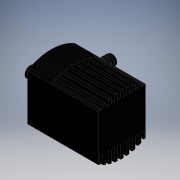
# Autodesk Inventor part: To Much Work, Motor
Saved by Autodesk Inventor 2016 (Build 200138000, 138)
## iProperties
Created: 2016-03-05
Part Number: To Much Work, Motor
Material: Generic
Document SubType Name: Modeling
Designer: Kenneth Daniel
Density: 1 g/cm^3
Appearance: Default
Author: Kenneth Daniel
Autodesk Inventor part; units mm, degrees
ref_plane "YZ Plane" through (0, 0, 0) normal (1, 0, 0) x (0, 1, 0)
ref_plane "XZ Plane" through (0, 0, 0) normal (0, 1, 0) x (-1, 0, 0)
sketch "Sketch1" plane through (0, 0, 0) normal (0, 1, 0) x (-1, 0, 0)
  line L0 (25.5, -21.35) -> (-25.5, -21.35)
  line L1 (-25.5, -21.35) -> (-25.5, 21.35)
  line L2 (-25.5, 21.35) -> (25.5, 21.35)
  line L3 (25.5, 21.35) -> (25.5, -21.35)
  line L4 (25.5, -21.35) -> (-25.5, 21.35) construction
  line L5 (-25.5, -21.35) -> (25.5, 21.35) construction
  point P0 (0, 0)
  dimension "d0" = 51
  dimension "d1" = 42.7
  constraints: 12 end point, 2 midpoint, 2 parallel, 1 horizontal, 1 perpendicular
  measures "d0" distance of L0.start L0.end
  measures "d1" distance of L0.end L1.end
extrude "Extrusion1" add sketch "Sketch1" along normal blind 34
sketch "Sketch2" plane through (-25.5, 0, -21.35) normal (-1, 0, 0) x (0, 0, 1)
  line L0 (42.7, 0) -> (0, 0) projected
  line L1 (42.7, 0) -> (42.7, 34) projected
  line L2 (0, 34) -> (42.7, 34) projected
  line L3 (0, 0) -> (0, 34) projected
  arc A0 (38.0522, 0) -> (38.0522, 34) centre (9.2864, 17) ccw
  line L4 (0, 34) -> (42.7, 34) construction
  line L5 (21.35, 34) -> (21.35, 0) construction
  arc A1 (4.6478, 34) -> (4.6478, 0) centre (33.4136, 17) ccw
  line L6 (0, 17) -> (42.7, 17) construction
  line L7 (42.7, 0) -> (0, 0) construction
  line L8 (9.5522, 34) -> (9.5522, 0) construction
  line L9 (9.5522, 34) -> (9.5522, 0)
  line L10 (0, 0) -> (0, 34) construction
  line L11 (0.0169, 18.0624) -> (9.5522, 18.0624) construction
  line L12 (9.5522, 15.937) -> (0, 15.937) construction
  line L13 (9.5522, 18.0624) -> (0.0169, 18.0624)
  line L14 (9.5522, 15.937) -> (0.0169, 15.937)
  line L15 (0.152, 20.1831) -> (9.5522, 20.1831)
  line L16 (0.4243, 22.3081) -> (9.5522, 22.3081)
  line L17 (0.8373, 24.4331) -> (9.5522, 24.4331)
  line L18 (1.3962, 26.5581) -> (9.5522, 26.5581)
  line L19 (2.1091, 28.6831) -> (9.5522, 28.6831)
  line L20 (2.9865, 30.8081) -> (9.5522, 30.8081)
  line L21 (4.0434, 32.9331) -> (9.5522, 32.9331)
  line L22 (0.1524, 13.812) -> (9.5522, 13.812)
  line L23 (0.4251, 11.687) -> (9.5522, 11.687)
  line L24 (0.8384, 9.562) -> (9.5522, 9.562)
  line L25 (1.3977, 7.437) -> (9.5522, 7.437)
  line L26 (2.1109, 5.312) -> (9.5522, 5.312)
  line L27 (2.9888, 3.187) -> (9.5522, 3.187)
  line L28 (4.0461, 1.062) -> (9.5522, 1.062)
  line L29 (9.5522, 34) -> (0, 34)
  line L30 (0, 34) -> (0, 0)
  line L31 (0, 0) -> (4.6478, 0)
  line L32 (42.7, 0) -> (42.7, 34) projected
  line L33 (42.7, 0) -> (42.7, 34)
  line L34 (42.7, 34) -> (9.5522, 34)
  line L35 (42.7, 0) -> (0, 0)
  line L36 (4.6478, 34) -> (4.0434, 32.9331)
  dimension "d4" = 28.5
  dimension "d5" = 1.0625
  dimension "d6" = 1.063
  dimension "d7" = 2.125
  dimension "d8" = 2.125
  dimension "d9" = 2.125
  dimension "d10" = 2.125
  dimension "d11" = 2.125
  dimension "d12" = 2.125
  dimension "d13" = 2.125
  dimension "d14" = 2.125
  dimension "d15" = 2.125
  dimension "d16" = 2.125
  dimension "d17" = 2.125
  dimension "d18" = 2.125
  dimension "d19" = 2.125
  dimension "d20" = 2.125
  dimension "d21" = 1.062
  dimension "d22" = 1.0669
  constraints: 56 end point, 9 perpendicular, 6 collinear, 6 horizontal, 5 point on line, 4 parallel, 3 point on circle, 3 symmetric about line, 2 vertical, 1 centre point, 1 midpoint, 41 other
  measures "d4" distance of A0.end L8.start
  measures "d5" distance of L6.start L11.start
  measures "d6" distance of L6.start L12.end
  measures "d7" distance of L15.start L11.start
  measures "d8" distance between parallel lines of L16 L15
  measures "d9" distance between parallel lines of L17 L16
  measures "d10" distance between parallel lines of L18 L17
  measures "d11" distance between parallel lines of L19 L18
  measures "d12" distance between parallel lines of L20 L19
  measures "d13" distance between parallel lines of L21 L20
  measures "d14" distance between parallel lines of L22 L12
  measures "d15" distance between parallel lines of L23 L22
  measures "d16" distance between parallel lines of L24 L23
  measures "d17" distance between parallel lines of L25 L24
  measures "d18" distance between parallel lines of L26 L25
  measures "d19" distance between parallel lines of L27 L26
  measures "d20" distance between parallel lines of L28 L27
  measures "d21" distance of L8.end L28.end
  measures "d22" distance of L21.end L8.start
extrude "Extrusion2" cut sketch "Sketch2" against normal through all contours L0 L3 A1 | L28 A1 L27 L9 | L9 L21 L36 L2 | A1 L3 L2 | L9 L20 A1 L21 | L26 A1 L25 L9 | A1 L15 L9 L13 | L14 L9 L22 A1 | L9 L18 A1 L19 | L24 A1 L23 L9 | A1 L17 L9 L16
sketch "Sketch3" plane through (-25.5, 0, 21.35) normal (-1, 0, 0) x (0, 0, 1)
  line L0 (-38.6566, 32.9331) -> (-33.1478, 32.9331)
  line L1 (-33.1478, 34) -> (-33.1478, 30.8081) projected
  line L2 (0, 34) -> (-33.1478, 34) projected
  line L3 (-38.0522, 34) -> (-33.1478, 34)
  line L4 (-33.1478, 34) -> (-33.1478, 32.9331)
  arc A0 (-38.0522, 34) -> (-38.6566, 32.9331) centre (-9.2864, 17) ccw projected
  line L5 (-38.0522, 34) -> (-38.0522, 34)
  line L6 (-38.0522, 34) -> (-38.6566, 32.9331)
  point P0 (-21.35, 0)
  constraints: 10 end point, 2 horizontal, 2 point on line, 1 collinear, 1 point on circle
extrude "Extrusion3" add sketch "Sketch3" against normal blind 51 contours L6 L3 L1 L0
sketch "Sketch4" plane through (-25.5, 0, 21.35) normal (0, 0, 1) x (1, 0, 0)
  line L0 (51, 34) -> (0, 34) projected
  line L1 (17, 34) -> (17, 0)
  line L2 (0, 0) -> (51, 0) projected
  line L3 (0, 30.8081) -> (51, 30.8081) projected
  line L4 (0, 28.6831) -> (51, 28.6831) projected
  line L5 (0, 26.5581) -> (51, 26.5581) projected
  line L6 (0, 24.4331) -> (51, 24.4331) projected
  line L7 (0, 22.3081) -> (51, 22.3081) projected
  line L8 (0, 20.1831) -> (51, 20.1831) projected
  line L9 (0, 18.0624) -> (51, 18.0624) projected
  line L10 (51, 15.937) -> (0, 15.937) projected
  line L11 (51, 0) -> (0, 0) projected
  line L12 (51, 0) -> (51, 34) projected
  line L13 (0, 34) -> (51, 34) projected
  line L14 (0, 0) -> (0, 34) projected
  line L15 (0, 13.812) -> (51, 13.812) projected
  line L16 (0, 11.687) -> (51, 11.687) projected
  line L17 (0, 9.562) -> (51, 9.562) projected
  line L18 (0, 7.437) -> (51, 7.437) projected
  line L19 (0, 5.312) -> (51, 5.312) projected
  line L20 (0, 3.187) -> (51, 3.187) projected
  line L21 (0, 1.062) -> (51, 1.062) projected
  line L22 (0, 32.9331) -> (51, 32.9331) projected
  line L23 (17, 34) -> (51, 34)
  line L24 (51, 34) -> (51, 0)
  line L25 (51, 1.062) -> (51, 3.187) projected
  line L26 (51, 0) -> (51, 1.062) projected
  line L27 (51, 0) -> (17, 0)
  line L28 (17, 1.062) -> (51, 1.062)
  line L29 (51, 3.187) -> (51, 5.312) projected
  line L30 (51, 3.187) -> (17, 3.187)
  line L31 (17, 5.312) -> (51, 5.312)
  line L32 (51, 5.312) -> (51, 7.437)
  line L33 (51, 7.437) -> (17, 7.437)
  line L34 (51, 7.437) -> (51, 9.562) projected
  line L35 (17, 9.562) -> (51, 9.562)
  line L36 (51, 9.562) -> (51, 11.687)
  line L37 (51, 11.687) -> (51, 13.812) projected
  line L38 (17, 11.687) -> (51, 11.687)
  line L39 (51, 11.687) -> (51, 13.812)
  line L40 (51, 13.812) -> (17, 13.812)
  line L41 (0, 13.812) -> (51, 13.812) projected
  line L42 (0, 15.937) -> (51, 15.937) projected
  line L43 (51, 15.937) -> (51, 18.0624) projected
  line L44 (17, 15.937) -> (51, 15.937)
  line L45 (51, 15.937) -> (51, 18.0624)
  line L46 (51, 18.0624) -> (17, 18.0624)
  line L47 (17, 20.1831) -> (51, 20.1831)
  line L48 (51, 22.3081) -> (17, 22.3081)
  line L49 (17, 24.4331) -> (51, 24.4331)
  line L50 (51, 26.5581) -> (17, 26.5581)
  line L51 (0, 26.5581) -> (51, 26.5581) projected
  line L52 (51, 28.6831) -> (51, 30.8081) projected
  line L53 (17, 28.6831) -> (51, 28.6831)
  line L54 (51, 28.6831) -> (51, 30.8081)
  line L55 (51, 30.8081) -> (17, 30.8081)
  line L56 (51, 30.8081) -> (51, 32.9331) projected
  line L57 (17, 32.9331) -> (51, 32.9331)
  point P0 (25.5, 0)
  dimension "d27" = 17
  constraints: 48 end point, 18 point on line, 7 collinear, 5 horizontal, 3 perpendicular, 2 vertical, 21 other
  measures "d27" distance of L23.start L0.end
extrude "Extrusion4" cut sketch "Sketch2" against normal blind 51 contours L0 A0 L1 | A0 L2 L1
sketch "Sketch5" plane through (25.5, 18.0624, -11.7978) normal (1, 0, 0) x (0, 0, -1)
  arc A0 (-28.5, 15.9376) -> (-28.5, -18.0624) centre (0.2657, -1.0624) ccw projected
  line L0 (-28.5, -18.0624) -> (-28.5, 15.9376)
  line L1 (-33.1478, -18.0624) -> (-33.1478, 15.9376) projected
  line L2 (-29.1017, -17.0004) -> (-28.5, -17.0004)
  line L3 (-30.1591, -14.8754) -> (-28.5, -14.8754)
  line L4 (-31.037, -12.7504) -> (-28.5, -12.7504)
  line L5 (-31.7501, -10.6254) -> (-28.5, -10.6254)
  line L6 (-32.3095, -8.5004) -> (-28.5, -8.5004)
  line L7 (-32.7227, -6.3754) -> (-28.5, -6.3754)
  line L8 (-32.9954, -4.2504) -> (-28.5, -4.2504)
  line L9 (-33.1309, -2.1254) -> (-28.5, -2.1254)
  line L10 (-33.131, 0) -> (-28.5, 0)
  line L11 (-32.9959, 2.1207) -> (-28.5, 2.1207)
  line L12 (-32.7235, 4.2457) -> (-28.5, 4.2457)
  line L13 (-32.3106, 6.3707) -> (-28.5, 6.3707)
  line L14 (-31.7516, 8.4957) -> (-28.5, 8.4957)
  line L15 (-31.0388, 10.6207) -> (-28.5, 10.6207)
  line L16 (-30.1613, 12.7457) -> (-28.5, 12.7457)
  line L17 (-29.1044, 14.8707) -> (-28.5, 14.8707)
  line L18 (-33.131, 0) -> (-28.5, 0)
  line L19 (-33.131, 0) -> (-28.5, 0)
  point P0 (-11.7978, -18.0624)
  point P1 (-33.1478, -12.7504)
  point P2 (-33.1478, -10.6254)
  point P3 (-33.1478, -8.5004)
  point P4 (-33.1478, -6.3754)
  point P5 (-33.1478, -4.2504)
  point P6 (-33.1478, -2.1254)
  point P7 (-33.1478, 0)
  point P8 (-33.1478, 2.1207)
  point P9 (-33.1478, 4.2457)
  point P10 (-33.1478, 6.3707)
  point P11 (-33.1478, 8.4957)
  point P12 (-33.1478, 10.6207)
  point P13 (-33.1478, 12.7457)
  point P14 (-33.1478, 14.8707)
  point P15 (-33.1478, -14.8754)
  point P16 (-33.1478, -17.0004)
  constraints: 36 end point, 15 horizontal, 2 collinear, 1 parallel, 37 other
extrude "Extrusion5" cut sketch "Sketch5" against normal blind 34 contours L17 L0 L16 A0 | L15 L0 L14 A0 | L13 L0 L12 A0 | L11 L0 L10 A0 | L0 L8 A0 L9 | L0 L6 A0 L7 | L0 L4 A0 L5 | L0 L2 A0 L3
sketch "Sketch6" plane through (0, 34, 0) normal (0, 1, 0) x (1, 0, 0)
  line L0 (-25.5, 16.7022) -> (25.5, 16.7022) construction
  line L1 (-18.54, 16.7022) -> (-18.54, -16.7022) construction
  line L2 (25.5, -16.7022) -> (-25.5, -16.7022) construction
  line L3 (-25.5, 16.7022) -> (-25.5, -16.7022) construction
  circle A0 centre (-18.54, 0) radius 3.9688 construction
  circle A1 centre (-18.54, 0) radius 5.5563 construction
  circle A2 centre (-18.54, 0) radius 3.5 construction
  circle A3 centre (-18.54, 0) radius 3.5
  circle A4 centre (-18.54, 0) radius 3.9688
  point P0 (0, 0)
  dimension "d32" = 6.96
  dimension "d33" = 7.9375
  dimension "d34" = 11.1125
  dimension "d35" = 7
  constraints: 5 centre point, 4 coincident, 2 end point, 2 point on line, 1 concentric, 1 midpoint, 1 vertical
  measures "d32" distance between parallel lines of L3 L1
  measures "d33" diameter of A0
  measures "d34" diameter of A1
  measures "d35" diameter of A2
extrude "Extrusion6" add sketch "Sketch6" along normal blind 20
ref_plane "Work Plane3" through (-18.54, 34, 0) normal (0, 0, -1) x (-1, 0, 0)
ref_plane "Work Plane1" through (-18.54, 34, 3.9688) normal (0, 0, -1) x (-1, 0, 0)
ref_plane "Work Plane2" through (-18.54, 34, -3.9688) normal (0, 0, -1) x (-1, 0, 0)
sketch "Sketch7" plane through (-18.54, 34, 0) normal (0, 0, -1) x (-1, 0, 0)
  line L0 (3.9688, 20) -> (-3.9688, 20) projected
  line L1 (-3.9688, 0) -> (3.9688, 0) projected
  line L2 (3.9688, 20) -> (-3.9688, 20) projected
  line L3 (-3.9688, 0) -> (3.9688, 0) projected
  line L4 (3.9688, 20) -> (-3.9688, 20) projected
  line L5 (3.5, 0) -> (3.5, 20) projected
  line L6 (3.5, 17.4442) -> (3.9688, 17.4442)
  arc A0 (3.9688, 18.1132) -> (3.5, 20) centre (-1.4093, 17.7787) ccw
  line L7 (3.9688, 0) -> (3.9688, 20) projected
  line L8 (3.9688, 18.1132) -> (3.5, 17.4442)
  line L9 (3.9688, 17.4442) -> (2.7369, 17.4442) construction
  arc A1 (3.9688, 15.5575) -> (3.5, 17.4442) centre (-1.4093, 15.2229) ccw
  line L10 (3.9688, 15.5575) -> (3.5, 14.8884)
  arc A2 (3.9688, 13.0017) -> (3.5, 14.8884) centre (-1.4093, 12.6671) ccw
  line L11 (3.9688, 13.0017) -> (3.5, 12.3326)
  arc A3 (3.9688, 10.4459) -> (3.5, 12.3326) centre (-1.4093, 10.1113) ccw
  line L12 (3.9688, 10.4459) -> (3.5, 9.7768)
  line L13 (3.5, 20) -> (3.5, 9.7768) construction
  line L14 (0, 20) -> (0, 0) construction
  point P0 (-18.54, -34)
  dimension "d38" = 2.5558
  dimension "d39" = 0
  dimension "d40" = 0
  dimension "d41" = 0
  constraints: 16 end point, 8 point on circle, 4 centre point, 3 point on line, 2 midpoint, 1 collinear, 1 perpendicular
  measures "d38" distance between parallel lines of L0 L6
  measures "d39" distance of A2.end L10.end
  measures "d40" distance of L11.end A3.end
  measures "d41" distance of L6.start A1.end
revolve "Revolution1" cut sketch "Sketch7" angle 360 about axis through (-18.54, 54, 0) along (0, -1, 0) contours L7 A0 L0
sketch "Sketch8" plane through (-18.54, 34, 0) normal (0, 0, -1) x (-1, 0, 0)
  line L0 (-3.9688, 18.1132) -> (3.9688, 18.1132) projected
  line L1 (-3.9688, 18.1132) -> (-3.5, 17.5638)
  line L2 (-3.5, 0) -> (-3.5, 20) projected
  line L3 (-3.9688, 0) -> (-3.9688, 18.1132) projected
  arc A0 (-3.5, 17.5638) -> (-3.9688, 16.0073) centre (-0.6147, 15.846) ccw
  line L4 (-3.9688, 15.6848) -> (-3.5, 15.1353)
  arc A1 (-3.5, 15.1353) -> (-3.9688, 13.7438) centre (-0.9417, 13.4988) ccw
  line L5 (-3.9688, 13.2539) -> (-3.5, 12.7044)
  arc A2 (-3.5, 12.7044) -> (-3.9688, 11.1551) centre (-0.6356, 10.9922) ccw
  line L6 (-3.9688, 10.8293) -> (-3.5, 10.2798)
  line L7 (-3.5, 20) -> (3.5, 20) construction
  line L8 (0, 20) -> (0, 6.8356) construction
  point P0 (-18.54, -34)
  constraints: 10 end point, 6 point on circle, 4 point on line, 3 centre point, 1 midpoint, 1 vertical, 7 other
revolve "Revolution2" cut sketch "Sketch8" angle 360 about axis through (-18.54, 54, 0) along (0, -1, 0) contours L1 A0 L3 | A1 L3 L4 | A2 L3 L5
sketch "Sketch9" plane through (-25.5, 18.0624, -21.3331) normal (-1, 0, 0) x (0, 0, 1)
  line L0 (9.5353, 14.8707) -> (4.0266, 14.8707) construction
  line L1 (9.5353, 14.8707) -> (9.5353, 15.9376) construction
  line L2 (4.631, 15.9376) -> (38.0353, 15.9376) construction
  line L3 (9.5353, 15.9376) -> (38.0353, -18.0624) construction
  line L4 (38.0353, -18.0624) -> (38.0353, 15.9376) construction
  line L5 (38.0353, 14.8707) -> (38.0353, 12.7457) construction
  line L6 (38.0353, 15.9376) -> (9.5353, -18.0624) construction
  line L7 (38.0353, -18.0624) -> (4.631, -18.0624) construction
  circle A0 centre (21.3331, -1.0624) radius 3.5 construction
  circle A1 centre (21.3331, -1.0624) radius 3.969 construction
  circle A2 centre (21.3331, -1.0624) radius 3.5
  circle A3 centre (21.3331, -1.0624) radius 3.969
  point P0 (21.3331, -18.0624)
  dimension "d44" = 7
  dimension "d45" = 7.938
  constraints: 8 end point, 4 centre point, 3 coincident, 3 point on line, 2 concentric, 1 collinear, 1 vertical
  measures "d44" diameter of A0
  measures "d45" diameter of A1
extrude "Extrusion7" add sketch "Sketch9" along normal blind 15
sketch "Sketch10" plane through (-25.5, 18.0624, -21.3331) normal (-1, 0, 0) x (0, 0, 1)
  line L0 (9.5353, 14.8707) -> (4.0266, 14.8707) construction
  line L1 (9.5353, 14.8707) -> (9.5353, 15.9376) construction
  line L2 (4.631, 15.9376) -> (38.0353, 15.9376) construction
  line L3 (9.5353, 15.9376) -> (38.0353, -18.0624) construction
  line L4 (38.0353, -18.0624) -> (38.0353, 15.9376) construction
  line L5 (38.0353, 15.9376) -> (9.5353, -18.0624) construction
  line L6 (13.0353, 15.9376) -> (13.0353, -18.0624) construction
  line L7 (34.5353, 15.9376) -> (34.5353, -18.0624) construction
  circle A0 centre (13.0353, 11.7622) radius 1.75
  circle A1 centre (34.5353, 11.7622) radius 1.75
  circle A2 centre (34.5353, -13.8869) radius 1.75
  circle A3 centre (13.0353, -13.8869) radius 1.75
  point P0 (21.3331, -18.0624)
  dimension "d48" = 3.5
  dimension "d49" = 3.5
  dimension "d50" = 3.5
  dimension "d51" = 3.5
  dimension "d52" = 3.5
  dimension "d53" = 3.5
  constraints: 12 end point, 12 point on line, 4 centre point, 3 vertical, 1 parallel
  measures "d48" distance of L1.end L6.start
  measures "d49" distance of L2.end L7.start
  measures "d50" diameter of A0
  measures "d51" diameter of A1
  measures "d52" diameter of A2
  measures "d53" diameter of A3
extrude "Extrusion8" add sketch "Sketch10" along normal blind 0.75
body "Solid1"
